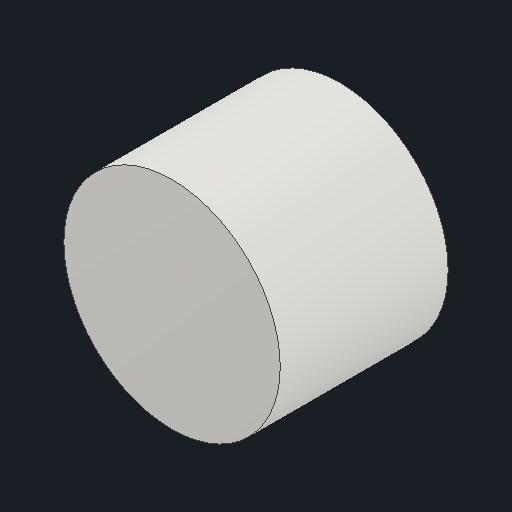
# Autodesk Inventor part: Шкив гладкий2
Saved by Autodesk Inventor 2024 (Build 280153000, 153)
## iProperties
Created: 2023-09-26
Part Number: Шкив гладкий2
Material: Steel
Document SubType Name: Modeling
Designer: user
Density: 7.85 g/cm^3
Appearance: Steel
CustomPartVersion: 1
Author: user
Autodesk Inventor part; units mm, degrees
ref_plane "YZ Plane" through (0, 0, 0) normal (1, 0, 0) x (0, 1, 0)
ref_plane "XZ Plane" through (0, 0, 0) normal (0, 1, 0) x (-1, 0, 0)
ref_plane "XY Plane" through (0, 0, 0) normal (0, 0, 1) x (1, 0, 0)
sketch "Основной эскиз" plane through (0, 0, 0) normal (0, 0, 1) x (1, 0, 0)
  circle A0 centre (0, 0) radius 4.5
  dimension "d0" = 9
  constraints: 1 centre point, 1 coincident
  measures "d0" diameter of A0
extrude "Шкив" add sketch "Основной эскиз" along normal mid plane 6.985
equation "\"d0\" = da_D"
equation "\"d1\" = da_B"
equation "\"da_D\" = 9"
equation "\"da_B\" = 6.985"
body "Solid1"
